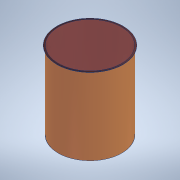
# Autodesk Inventor part: smietnik1_srodek
Saved by Autodesk Inventor 2021 (Build 250183000, 183)
## iProperties
Created: 2025-11-29
Part Number: smietnik1_srodek
Material: Generic
Document SubType Name: Modeling
Designer: huber
Density: 1 g/cm^3
Appearance: Cool Tint
Author: huber
Autodesk Inventor part; units mm, degrees
ref_plane "YZ Plane" through (0, 0, 0) normal (1, 0, 0) x (0, 1, 0)
ref_plane "XZ Plane" through (0, 0, 0) normal (0, 1, 0) x (-1, 0, 0)
ref_plane "XY Plane" through (0, 0, 0) normal (0, 0, 1) x (1, 0, 0)
sketch "Sketch1" plane through (0, 0, 0) normal (1, 0, 0) x (0, 1, 0)
  line L0 (0, 0) -> (0, 255)
  line L1 (0, 255) -> (620, 255)
  line L2 (620, 255) -> (620, 265)
  line L3 (-124, 0) -> (744, 0) projected
  dimension "d0" = 620
  dimension "d1" = 255
  dimension "d2" = 10
  constraints: 6 end point, 2 perpendicular, 1 vertical
  measures "d0" distance of L0.end L1.end
  measures "d1" distance of L0.start L0.end
  measures "d2" distance of L1.end L2.end
surface revolve "RevolutionSrf1" sketch "Sketch1" angle 360 about axis through (0, -10, 0) along (0, 1, 0) shown yes curves L0 L1 L2
thicken "Thicken1" operation new thickness 2 both sides no extend neighbours no toward (0.0589628, 0, -0.9982602) faces at (-15.0355, 413.3333, 254.5563) (258.1049, 620, 5.6577) (70.5152, 0, 40.8296)
body "Solid1"
body "Srf1"
